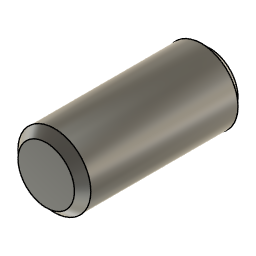
shaft (Autodesk Fusion 360 design; units mm, degrees)
Autodesk Fusion 360 part; units mm, degrees
sketch "Sketch1" plane through (0, 0, 0) normal (0, 1, 0) x (1, 0, 0)
  circle A0 centre (0, 0) radius 4.45
  dimension "d1" = 8.9
  constraint coincident A0.centre origin
  measures "d1" diameter of A0
extrude "Extrude1" add sketch "Sketch1" along normal blind 20
chamfer "Chamfer1" distance 1 angle 45 2 edges at (-4.1489, 0, 1.6092) (-4.1489, 20, 1.6092)
